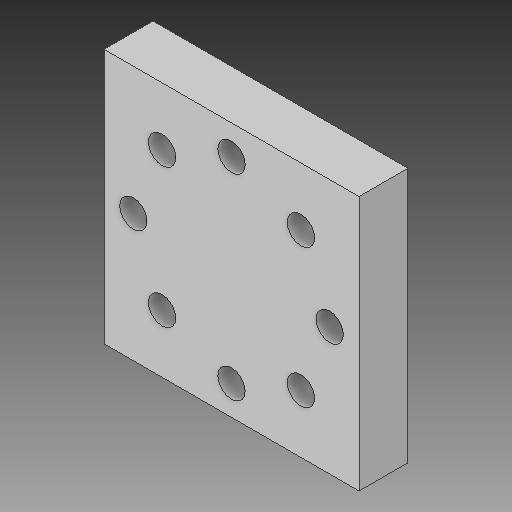
# Autodesk Inventor part: GlyphtPlateAttachment
Saved by Autodesk Inventor 2017 (Build 210142000, 142)
## iProperties
Created: 2018-01-10
Part Number: GlyphtPlateAttachment
Material: Generic
Document SubType Name: Modeling
Designer: User
Density: 1 g/cm^3
Appearance: Default
Author: User
Autodesk Inventor part; units mm, degrees
ref_plane "YZ Plane" through (0, 0, 0) normal (1, 0, 0) x (0, 1, 0)
ref_plane "XZ Plane" through (0, 0, 0) normal (0, 1, 0) x (-1, 0, 0)
ref_plane "XY Plane" through (0, 0, 0) normal (0, 0, 1) x (1, 0, 0)
sketch "Sketch1" plane through (0, 0, 0) normal (0, 0, 1) x (1, 0, 0)
  line L0 (0, 0) -> (25.4, 0)
  line L1 (25.4, 0) -> (25.4, -25.4)
  line L2 (25.4, -25.4) -> (0, -25.4)
  line L3 (0, -25.4) -> (0, 0)
  dimension "d0" = 25.4
  dimension "d1" = 25.4
  constraints: 8 end point, 2 parallel, 1 horizontal, 1 perpendicular
  measures "d0" distance of L1.end L2.end
  measures "d1" distance of L0.end L1.end
extrude "Extrusion1" add sketch "Sketch1" along normal blind 4.8768
sketch "Sketch2" plane through (0, 0, 4.8768) normal (0, 0, 1) x (1, 0, 0)
  line L0 (0, 0) -> (0, -25.4) projected
  line L1 (0, -12.7) -> (12.7, -12.7)
  line L2 (12.7, -12.7) -> (12.7, -2.921)
  point P0 (5.7852, -5.7852)
  point P1 (2.921, -12.7)
  point P2 (5.7852, -19.6148)
  point P3 (12.7, -22.479)
  point P4 (19.6148, -19.6148)
  point P5 (22.479, -12.7)
  point P6 (19.6148, -5.7852)
  dimension "d4" = 12.7
  dimension "d5" = 9.779
  dimension "d15" = 360
  constraints: 4 end point, 1 coincident, 1 horizontal, 1 midpoint, 1 perpendicular, 9 other
  measures "d4" distance of L1.start L1.end
  measures "d5" distance of L1.end L2.end
hole "Hole1" at (12.7, -2.921, 4.8768) at (19.6148, -5.7852, 4.8768) at (22.479, -12.7, 4.8768) at (19.6148, -19.6148, 4.8768) at (12.7, -22.479, 4.8768) at (5.7852, -19.6148, 4.8768) at (2.921, -12.7, 4.8768) at (5.7852, -5.7852, 4.8768) direction (0, 0, -1) diameter 2.7178 depth 25.4 tip angle 118
sketch "Sketch3" plane through (0, 0, 4.8768) normal (0, 0, 1) x (1, 0, 0)
  point P0 (0, 0)
body "Solid1"
